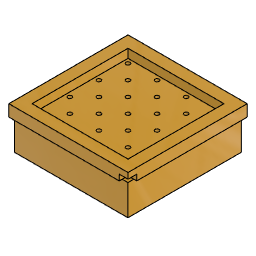
Silicon_moulds (Autodesk Fusion 360 design; units mm, degrees)
Autodesk Fusion 360 part; units mm, degrees
sketch "Sketch1" plane through (0, 0, 0) normal (0, 0, 1) x (1, 0, 0)
  line L0 (20, 20) -> (-20, 20)
  line L1 (-20, 20) -> (-20, -20)
  line L2 (-20, -20) -> (20, -20)
  line L3 (20, -20) -> (20, 20)
  line L4 (20, 20) -> (-20, -20) construction
  line L5 (-20, 20) -> (20, -20) construction
  dimension "d1" = 40
  dimension "d2" = 40
  constraint horizontal L0
  constraint perpendicular L0 L1
  constraint parallel L0 L2
  constraint parallel L1 L3
  constraint coincident L4 origin
  constraint coincident L5 origin
  measures "d1" distance of L1.end L2.end
  measures "d2" distance of L0.end L1.end
sketch "Sketch2" plane through (0, 0, 10) normal (0, 0, 1) x (-1, 0, 0)
sketch "Sketch3" plane through (0, 0, 0) normal (0, 0, 1) x (1, 0, 0)
  line L0 (20.5, 20.5) -> (-20.5, 20.5)
  line L1 (-20.5, 20.5) -> (-20.5, -20.5)
  line L2 (-20.5, -20.5) -> (20.5, -20.5)
  line L3 (20.5, -20.5) -> (20.5, 20.5)
  line L4 (20.5, 20.5) -> (-20.5, -20.5) construction
  line L5 (-20.5, 20.5) -> (20.5, -20.5) construction
  dimension "d7" = 41
  dimension "d8" = 41
  constraint horizontal L0
  constraint perpendicular L0 L1
  constraint parallel L0 L2
  constraint parallel L1 L3
  constraint coincident L4 origin
  constraint coincident L5 origin
  measures "d7" distance of L1.end L2.end
  measures "d8" distance of L0.end L1.end
extrude "Extrude2" add sketch "Sketch3" along normal blind 11 makes body 1
sketch "Sketch4" plane through (0, 0, 11) normal (0, 0, 1) x (-1, 0, 0)
  line L0 (-20.5, 20.5) -> (-20.5, -20.5)
  line L1 (-20.5, -20.5) -> (20.5, -20.5)
  line L2 (20.5, -20.5) -> (20.5, 20.5)
  line L3 (20.5, 20.5) -> (-20.5, 20.5)
  line L4 (-15, -15) -> (15, -15)
  line L5 (15, -15) -> (15, 15)
  line L6 (15, 15) -> (-15, 15)
  line L7 (-15, 15) -> (-15, -15)
  line L8 (-15, -15) -> (15, 15) construction
  line L9 (15, -15) -> (-15, 15) construction
  dimension "d11" = 30
  dimension "d12" = 30
  constraint horizontal L4
  constraint perpendicular L4 L5
  constraint parallel L4 L6
  constraint parallel L5 L7
  constraint coincident L8 origin
  constraint coincident L9 origin
  measures "d11" distance of L5.end L6.end
  measures "d12" distance of L4.end L5.end
extrude "Extrude3" cut sketch "Sketch4" against normal blind 9 contours L4 L5 L6 L7 bodies 1
draft "Draft1" angle 9.46 neutral plane through (0, 0, 2) pull (0, 0, 1) 1 faces at (-15, 5, 8) on bodies 1
draft "Draft2" angle 9.46 neutral plane through (0, 0, 2) pull (0, 0, 1) 1 faces at (-5.4999, -15, 8) on bodies 1
draft "Draft3" angle 9.46 neutral plane through (0, 0, 2) pull (0, 0, 1) 1 faces at (15, -5.4999, 8) on bodies 1
draft "Draft4" angle 9.46 neutral plane through (0, 0, 2) pull (0, 0, 1) 1 faces at (-5, 15, 8) on bodies 1
sketch "Sketch5" plane through (0, 0, 2) normal (0, 0, 1) x (-1, 0, 0)
  line L0 (-15, 15) -> (-15, -15)
  line L1 (-15, -15) -> (15, -15)
  line L2 (15, -15) -> (15, 15)
  line L3 (15, 15) -> (-15, 15)
  circle A0 centre (3.25, 3.25) radius 1.05
  dimension "d23" = 2.1
  measures "d23" diameter of A0
extrude "Extrude4" add sketch "Sketch5" along normal blind 1.1 contours A0 bodies 1
sketch "Sketch6" plane through (0, 0, 2) normal (0, 0, 1) x (-1, 0, 0)
  circle A0 centre (3.25, 3.25) radius 1.05
  line L0 (-15, 15) -> (-15, -15)
  line L1 (-15, -15) -> (15, -15)
  line L2 (15, -15) -> (15, 15)
  line L3 (15, 15) -> (-15, 15)
  circle A1 centre (15, 15) radius 10
  dimension "d26" = 20
  constraint coincident L2.end L3.start
  measures "d26" diameter of A1
extrude "Extrude5" add sketch "Sketch6" along normal blind 5 contours L2 L3 A1 | L2 L3 A1 bodies 1
delete_face "DeleteFace1" 1 faces at (-7.23, -21.295, 3.6667) on bodies 1
sketch "Sketch7" plane through (0, 0, 0) normal (0, 0, 1) x (1, 0, 0)
  line L0 (-16.4995, 16.4995) -> (16.4995, 16.4995)
  line L1 (16.4995, 16.4995) -> (16.4995, -16.4995)
  line L2 (16.4995, -16.4995) -> (-16.4995, -16.4995)
  line L3 (-16.4995, -16.4995) -> (-16.4995, 16.4995)
  line L4 (-16.4995, 16.4995) -> (16.4995, -16.4995) construction
  line L5 (16.4995, 16.4995) -> (-16.4995, -16.4995) construction
  dimension "d29" = 32.999
  dimension "d30" = 32.999
  constraint horizontal L0
  constraint perpendicular L0 L1
  constraint parallel L0 L2
  constraint parallel L1 L3
  constraint coincident L4 origin
  constraint coincident L5 origin
  measures "d29" distance of L1.end L2.end
  measures "d30" distance of L0.end L1.end
extrude "Extrude6" add sketch "Sketch7" along normal blind 4 separate body makes body 2
draft "Draft5" angle -9.46 neutral plane through (0, 0, 4) pull (0, 0, 1) 1 faces at (16.4995, 5.4998, 1.3333) on bodies 2
draft "Draft6" angle -9.46 neutral plane through (0, 0, 4) pull (0, 0, 1) 1 faces at (5.2777, 16.4995, 2.6667) on bodies 2
draft "Draft7" angle -9.46 neutral plane through (0, 0, 4) pull (0, 0, 1) 1 faces at (-16.4995, 5.2777, 2.6667) on bodies 2
draft "Draft8" angle -9.46 neutral plane through (0, 0, 4) pull (0, 0, 1) 1 faces at (5.2777, -16.4995, 2.6667) on bodies 2
sketch "Sketch8" plane through (0, 0, 4) normal (0, 0, 1) x (-1, 0, 0)
  line L0 (16.4995, 16.4995) -> (-16.4995, 16.4995)
  line L1 (-16.4995, 16.4995) -> (-16.4995, -16.4995)
  line L2 (-16.4995, -16.4995) -> (16.4995, -16.4995)
  line L3 (16.4995, -16.4995) -> (16.4995, 16.4995)
  line L4 (-20.5, -20.5) -> (20.5, -20.5)
  line L5 (20.5, -20.5) -> (20.5, 20.5)
  line L6 (20.5, 20.5) -> (-20.5, 20.5)
  line L7 (-20.5, 20.5) -> (-20.5, -20.5)
  line L8 (-20.5, -20.5) -> (20.5, 20.5) construction
  line L9 (20.5, -20.5) -> (-20.5, 20.5) construction
  dimension "d41" = 41
  dimension "d42" = 41
  constraint horizontal L4
  constraint perpendicular L4 L5
  constraint parallel L4 L6
  constraint parallel L5 L7
  constraint coincident L8 origin
  constraint coincident L9 origin
  measures "d41" distance of L5.end L6.end
  measures "d42" distance of L4.end L5.end
extrude "Extrude7" add sketch "Sketch8" along normal blind 4 separate body makes body 3
combine "Combine1" operation add target body 2 tool bodies 3
sketch "Sketch9" plane through (0, 0, 4) normal (0, 0, 1) x (-1, 0, 0)
  line L0 (16.4995, 16.4995) -> (-16.4995, 16.4995)
  line L1 (-16.4995, 16.4995) -> (-16.4995, -16.4995)
  line L2 (-16.4995, -16.4995) -> (16.4995, -16.4995)
  line L3 (16.4995, -16.4995) -> (16.4995, 16.4995)
  circle A0 centre (10, -10) radius 0.7
  circle A1 centre (10, 0) radius 0.7
  circle A2 centre (10, 10) radius 0.7
  circle A3 centre (0, 0) radius 0.7
  circle A4 centre (0, -10) radius 0.7
  circle A5 centre (-10, -10) radius 0.7
  circle A6 centre (-10, 0) radius 0.7
  circle A7 centre (-10, 10) radius 0.7
  circle A8 centre (0, 10) radius 0.7
  circle A9 centre (5, 5) radius 0.7
  circle A10 centre (5, -5) radius 0.7
  circle A11 centre (-5, -5) radius 0.7
  circle A12 centre (-5, 5) radius 0.7
  dimension "d45" = 1.4
  dimension "d46" = 1.4
  dimension "d47" = 1.4
  dimension "d48" = 1.4
  dimension "d49" = 1.4
  dimension "d50" = 1.4
  dimension "d51" = 1.4
  dimension "d52" = 1.4
  dimension "d53" = 1.4
  dimension "d54" = 1.4
  dimension "d55" = 1.4
  dimension "d56" = 1.4
  dimension "d58" = 1.4
  constraint coincident A3.centre origin
  measures "d45" diameter of A0
  measures "d46" diameter of A1
  measures "d47" diameter of A2
  measures "d48" diameter of A3
  measures "d49" diameter of A4
  measures "d50" diameter of A5
  measures "d51" diameter of A6
  measures "d52" diameter of A7
  measures "d53" diameter of A8
  measures "d54" diameter of A9
  measures "d55" diameter of A10
  measures "d56" diameter of A11
  measures "d58" diameter of A12
extrude "Extrude8" cut sketch "Sketch9" against normal blind 4 contours A0 | A1 | A2 | A3 | A4 | A5 | A6 | A7 | A8 | A9 | A10 | A11 | A12 bodies 2
sketch "Sketch10" plane through (0, 0, 4) normal (0, 0, 1) x (-1, 0, 0)
  circle A0 centre (-10, -10) radius 0.7
  circle A1 centre (-5, 5) radius 0.7
  circle A2 centre (0, 0) radius 0.7
  circle A3 centre (5, -5) radius 0.7
  circle A4 centre (10, 10) radius 0.7
  circle A5 centre (0, -10) radius 0.7
  circle A6 centre (0, 10) radius 0.7
  circle A7 centre (-10, 0) radius 0.7
  circle A8 centre (5, 5) radius 0.7
  circle A9 centre (10, -10) radius 0.7
  circle A10 centre (10, 0) radius 0.7
  circle A11 centre (-5, -5) radius 0.7
  circle A12 centre (-10, 10) radius 0.7
  line L0 (16.4995, 16.4995) -> (-16.4995, 16.4995)
  line L1 (-16.4995, 16.4995) -> (-16.4995, -16.4995)
  line L2 (-16.4995, -16.4995) -> (16.4995, -16.4995)
  line L3 (16.4995, -16.4995) -> (16.4995, 16.4995)
  circle A13 centre (5, 15) radius 0.7
  circle A14 centre (-5, 15) radius 0.7
  circle A15 centre (-15, 5) radius 0.7
  circle A16 centre (-15, -5) radius 0.7
  circle A17 centre (-5, -15) radius 0.7
  circle A18 centre (-15, 15) radius 0.7
  circle A19 centre (-15, -15) radius 0.7
  circle A20 centre (5, -15) radius 0.7
  circle A21 centre (15, -15) radius 0.7
  circle A22 centre (15, -5) radius 0.7
  circle A23 centre (15, 5) radius 0.7
  circle A24 centre (15, 15) radius 0.7
  dimension "d61" = 1.4
  dimension "d62" = 1.4
  dimension "d63" = 1.4
  dimension "d64" = 1.4
  dimension "d65" = 1.4
  dimension "d66" = 1.4
  dimension "d67" = 1.4
  dimension "d68" = 1.4
  dimension "d69" = 1.4
  dimension "d70" = 1.4
  dimension "d71" = 1.4
  dimension "d72" = 1.4
  measures "d61" diameter of A13
  measures "d62" diameter of A14
  measures "d63" diameter of A15
  measures "d64" diameter of A16
  measures "d65" diameter of A17
  measures "d66" diameter of A18
  measures "d67" diameter of A19
  measures "d68" diameter of A20
  measures "d69" diameter of A21
  measures "d70" diameter of A22
  measures "d71" diameter of A23
  measures "d72" diameter of A24
extrude "Extrude9" cut sketch "Sketch10" against normal blind 4 contours A13 | A14 | A15 | A16 | A17 | A18 | A19 | A20 | A21 | A22 | A23 | A24 bodies 2
move_body "Move1" bodies 2 to x (1, 0, 0) y (0, 1, 0) z (0, 0, 1) at (0, 0, 7)
sketch "Sketch11" plane through (0, 0, 0) normal (1, 0, 0) x (0, 1, 0)
  line L0 (-20.5, 11, 20.5) -> (-17.5, 11, 20.5)
  line L1 (-17.5, 11, 20.5) -> (-17.5, 11, 17.5)
  line L2 (-17.5, 11, 17.5) -> (-20.5, 11, 17.5)
  line L3 (-20.5, 11, 17.5) -> (-20.5, 11, 20.5)
  point P0 (-20.5, 11)
  dimension "d75" = 3
extrude "Extrude10" cut sketch "Sketch11" along normal blind 2 contours L0 L1 L2 L3 in plane through (0, 0, 11) normal (0, 0, 1) bodies 2
sketch "Sketch12" plane through (0, 0, 11) normal (0, 0, -1) x (1, 0, 0)
  line L0 (20.5, 17.5) -> (17.5, 17.5)
  line L1 (17.5, 17.5) -> (17.5, 20.5)
  line L2 (17.5, 20.5) -> (-20.5, 20.5)
  line L3 (-20.5, 20.5) -> (-20.5, -20.5)
  line L4 (-20.5, -20.5) -> (20.5, -20.5)
  line L5 (20.5, -20.5) -> (20.5, 17.5)
  line L6 (-16.4995, -16.4995) -> (-16.4995, 16.4995)
  line L7 (-16.4995, 16.4995) -> (16.4995, 16.4995)
  line L8 (16.4995, 16.4995) -> (16.4995, -16.4995)
  line L9 (16.4995, -16.4995) -> (-16.4995, -16.4995)
  line L10 (-20.5, -20.5) -> (-17.5, -20.5)
  line L11 (-17.5, -20.5) -> (-17.5, -17.5)
  line L12 (-17.5, -17.5) -> (-20.5, -17.5)
  line L13 (-20.5, -17.5) -> (-20.5, -20.5)
  dimension "d78" = 3
  dimension "d79" = 3
  constraint horizontal L10
  constraint vertical L11
  constraint horizontal L12
  constraint vertical L13
  constraint coincident L3.end L4.start
  measures "d78" distance of L3.end L10.end
  measures "d79" distance of L3.end L12.end
extrude "Extrude11" cut sketch "Sketch12" against normal blind 2 contours L3 L4 L10 L11 L12 L13 bodies 2
draft "Draft9" angle 5 neutral plane through (0, 0, 2) pull (0, 0, 1) 1 faces at (-15.7776, 8.8216, 6.6667) on bodies 1
draft "Draft10" angle 5 neutral plane through (0, 0, 2) pull (0, 0, 1) 1 faces at (15.9998, -5, 8) on bodies 1
draft "Draft11" angle 5 neutral plane through (0, 0, 2) pull (0, 0, 1) 1 faces at (9.0869, -15.8647, 7.1893) on bodies 1
draft "Draft12" angle 5 neutral plane through (0, 0, 2) pull (0, 0, 1) 1 faces at (5, 15.9998, 8) on bodies 1
delete_face "DeleteFace2" 1 faces at (-14.1257, -5.0383, 4.0844) on bodies 1
sketch "Sketch13" plane through (0, 0, 2) normal (0, 0, 1) x (-1, 0, 0)
  line L0 (15, 15) -> (-15, 15)
  line L1 (-15, 15) -> (-15, -15)
  line L2 (-15, -15) -> (15, -15)
  line L3 (15, -15) -> (15, 15)
  circle A0 centre (3.25, 3.25) radius 1.05
  circle A1 centre (27, 14) radius 2.2361
extrude "Extrude12" add sketch "Sketch13" along normal blind 5 separate body contours A1 makes body 4
move_body "Move2" bodies 4 to x (1, 0, 0) y (0, 1, 0) z (0, 0, 1) at (11, -2, 0)
move_face "MoveFace1" by (-25.5968, -1.6567, 0) 1 faces at (-3.1133, -3.5175, 3.1) on bodies 1
sketch "Sketch14" plane through (0, 0, 2) normal (0, 0, 1) x (-1, 0, 0)
  line L0 (15, 15) -> (-15, 15)
  line L1 (-15, 15) -> (-15, -15)
  line L2 (-15, -15) -> (15, -15)
  line L3 (15, -15) -> (15, 15)
  circle A0 centre (3.25, 3.25) radius 1.05
  line L4 (13, -13) -> (10, -13)
  line L5 (10, -13) -> (10, 13)
  line L6 (10, 13) -> (13, 13)
  line L7 (13, 13) -> (13, -13)
  line L8 (10, -13) -> (-13, -13)
  line L9 (-13, -13) -> (-13, -10)
  line L10 (-13, -10) -> (10, -10)
  line L11 (10, -10) -> (10, -13)
  line L12 (10, 10) -> (-13, 10)
  line L13 (-13, 10) -> (-13, 13)
  line L14 (-13, 13) -> (10, 13)
  line L15 (10, 13) -> (10, 10)
  line L16 (-10, -10) -> (-13, -10)
  line L17 (-13, -10) -> (-13, 10)
  line L18 (-13, 10) -> (-10, 10)
  line L19 (-10, 10) -> (-10, -10)
  constraint horizontal L4
  constraint vertical L5
  constraint horizontal L6
  constraint vertical L7
  constraint horizontal L8
  constraint vertical L9
  constraint horizontal L10
  constraint vertical L11
  constraint horizontal L12
  constraint vertical L13
  constraint horizontal L14
  constraint vertical L15
  constraint coincident L5 L12.start
  constraint horizontal L16
  constraint vertical L17
  constraint horizontal L18
  constraint vertical L19
  constraint coincident L10 L16.start
extrude "Extrude13" cut sketch "Sketch14" against normal blind 0.5 contours L4 L5 L6 L7 L11 L15 | L5 L8 L9 L10 L11 L16 | L5 L12 L13 L14 L15 L18 | L10 L12 L16 L17 L18 L19 bodies 1
extrude "Extrude14" add 1 faces at (5.9178, -0.9802, 2) along direction (0, 0, 1) blind 0.8 on bodies 1 bodies 1
extrude "Extrude15" add 1 faces at (-3.1133, -3.5175, 3.1) along direction (0, 0, 1) blind 0.8 on bodies 1 bodies 1
extrude "Extrude16" add 1 faces at (5.9178, -0.9802, 2.8) along direction (0, 0, 1) blind 0.3 on bodies 1 bodies 1
extrude "Extrude17" add 1 faces at (-3.1133, -3.5175, 3.9) along direction (0, 0, 1) blind 0.3 on bodies 1 bodies 1
combine "Combine2" operation add target body 1 tool bodies 4
extrude "Extrude18" add 1 faces at (-13.6015, 10, 11) along direction (0, 0, 1) blind 1 on bodies 2 bodies 2
draft "Draft13" angle 5 neutral plane through (0, 0, 11) pull (0, 0, -1) 1 faces at (-5.2777, -16.2773, 9.6667) on bodies 2
draft "Draft14" angle 5 neutral plane through (0, 0, 11) pull (0, 0, -1) 1 faces at (-16.2773, -5.156, 9.6667) on bodies 2
draft "Draft15" angle 5 neutral plane through (0, 0, 11) pull (0, 0, -1) 1 faces at (-5.156, 16.2773, 9.6667) on bodies 2
draft "Draft16" angle 5 neutral plane through (0, 0, 11) pull (0, 0, -1) 1 faces at (16.2773, -5.156, 9.6667) on bodies 2
scale "Scale1" factor 1.02 about (-20.5, 17.5, 11) bodies 2
scale "Scale2" factor 1.02 about (-3.976, 4.75, 12.02) bodies 2
move_body "Move3" bodies 2 to x (1, 0, 0) y (0, 1, 0) z (0, 0, 1) at (-0.5, 0, 0)
scale "Scale3" factor 1.01 about (5.928, 4.75, 12.02) bodies 2
move_body "Move4" bodies 1 to x (1, 0, 0) y (0, 1, 0) z (0, 0, 1) at (-0.1, -0.5, -0.05)
named bodies: "button", "lid"
